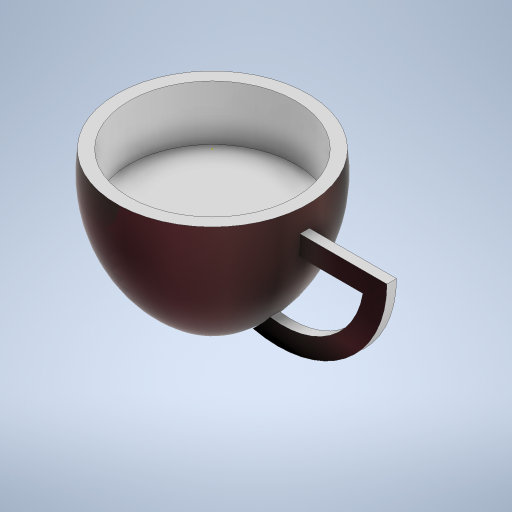
# Autodesk Inventor part: practice
Saved by Autodesk Inventor 2024 (Build 280153000, 153)
## iProperties
Created: 2024-02-20
Part Number: practice
Material: Generic
Document SubType Name: Modeling
Designer: HP
Density: 1 g/cm^3
Appearance: Default
Author: HP
Autodesk Inventor part; units mm, degrees
ref_plane "YZ Plane" through (0, 0, 0) normal (1, 0, 0) x (0, 1, 0)
ref_plane "XZ Plane" through (0, 0, 0) normal (0, 1, 0) x (-1, 0, 0)
ref_plane "XY Plane" through (0, 0, 0) normal (0, 0, 1) x (1, 0, 0)
sketch "Sketch1" plane through (0, 0, 0) normal (0, 0, 1) x (1, 0, 0)
  line L0 (0, 0) -> (0, 14.749)
  line L1 (0, 14.749) -> (10.0027, 14.749)
  line L2 (0, 0) -> (3.1272, 0)
  line L3 (3.1272, 0) -> (4.2805, 0)
  arc A0 (3.1272, 0) -> (10.0027, 14.749) centre (-4.7238, 12.6369) ccw
  dimension "d0" = 3.1272
  constraints: 8 end point, 2 point on circle, 1 centre point, 1 perpendicular, 1 point on line, 1 vertical
  measures "d0" distance of L0.start L2.end
revolve "Revolution1" add sketch "Sketch1" angle 360 mid plane about axis through (0, 0, 0) along (0, 1, 0)
sketch "Sketch2" plane through (0, 14.749, 0) normal (0, 1, 0) x (1, 0, 0)
  point P0 (0, 0)
sketch "Sketch3" plane through (0, 0, 0) normal (0, 0, 1) x (1, 0, 0)
  arc A0 (3.1272, 0) -> (10.0027, 14.749) centre (-4.7238, 12.6369) ccw projected
  line L0 (10.0027, 10.5248) -> (16.7525, 10.5248)
  arc A1 (7.039, 3.5284) -> (16.7525, 10.5248) centre (8.3697, 11.9219) ccw
  line L1 (10.0027, 14.749) -> (10.0027, 10.5248)
  line L2 (10.0027, 12.6369) -> (19.2796, 12.6369)
  arc A2 (5.2442, 1.5929) -> (19.2796, 12.6369) centre (7.8732, 12.6923) ccw
  point P0 (0, 0)
  point P1 (10.1534, 12.6369)
  constraints: 8 point on circle, 6 end point, 2 centre point, 1 horizontal, 1 midpoint, 1 perpendicular, 1 vertical
extrude "Extrusion1" add sketch "Sketch3" along normal blind 1 contours A0 A1 L0 L2 A2
sketch "Sketch4" plane through (0, 14.749, 0) normal (0, 1, 0) x (1, 0, 0)
  circle A0 centre (0, 0) radius 8.7259
  constraints: 1 centre point, 1 coincident
extrude "Extrusion2" cut sketch "Sketch4" against normal blind 5.7625
sketch "Sketch5" plane through (0, 0, 0) normal (0, -1, 0) x (1, 0, 0)
  circle A0 centre (0, 0) radius 2.7204
  circle A1 centre (0, 0) radius 2.7204
  circle A2 centre (0, 0) radius 2.7204
  constraints: 3 centre point, 3 coincident, 1 concentric
extrude "Extrusion3" add sketch "Sketch5" along normal blind 0.1
sketch "Sketch6" plane through (0, 0, 0) normal (0, 0, 1) x (1, 0, 0)
  point P0 (0, 0)
sketch "Sketch7" plane through (0, 0, 0) normal (0, 0, 1) x (1, 0, 0)
  point P0 (0, 0)
sketch "Sketch8" plane through (0, 0, 0) normal (0, 0, 1) x (1, 0, 0)
  point P0 (0, 0)
body "Solid1"
